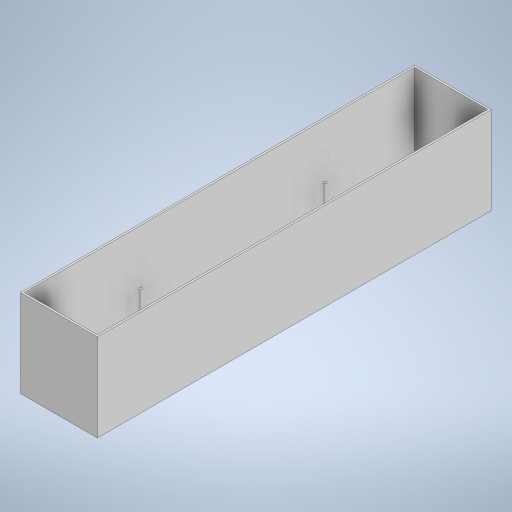
# Autodesk Inventor part: Box
Saved by Autodesk Inventor 2023 (Build 270158030, 158C)
## iProperties
Created: 2023-02-14
Part Number: Box
Material: Generic
Document SubType Name: Modeling
Designer: jeremyy
Density: 1 g/cm^3
Appearance: Default
Author: jeremyy
Autodesk Inventor part; units mm, degrees
ref_plane "YZ Plane" through (0, 0, 0) normal (1, 0, 0) x (0, 1, 0)
ref_plane "XZ Plane" through (0, 0, 0) normal (0, 1, 0) x (-1, 0, 0)
ref_plane "XY Plane" through (0, 0, 0) normal (0, 0, 1) x (1, 0, 0)
sketch "Sketch1" plane through (0, 0, 0) normal (0, 1, 0) x (-1, 0, 0)
  line L0 (0, 0) -> (127, 0)
  line L1 (127, 0) -> (127, -651.51)
  line L2 (127, -651.51) -> (0, -651.51)
  line L3 (0, -651.51) -> (0, 0)
  line L4 (123.825, -3.175) -> (3.175, -3.175)
  line L5 (3.175, -3.175) -> (3.175, -648.335)
  line L6 (3.175, -648.335) -> (123.825, -648.335)
  line L7 (123.825, -648.335) -> (123.825, -3.175)
  circle A0 centre (101.6, -478.155) radius 2.3812
  circle A1 centre (25.4, -478.155) radius 2.3813
  line L8 (3.175, -325.755) -> (14.531, -325.755)
  circle A2 centre (101.6, -173.355) radius 2.3812
  circle A3 centre (25.4, -173.355) radius 2.3813
  dimension "d0" = 127
  dimension "d1" = 651.51
  dimension "d2" = 3.175
  dimension "d13" = 4.7625
  dimension "d14" = 4.7625
  dimension "d15" = 76.2
  dimension "d16" = 25.4
  dimension "d17" = 152.4
  constraints: 18 end point, 4 centre point, 4 parallel, 2 horizontal, 2 perpendicular, 2 symmetric about line, 1 midpoint, 5 other
  measures "d0" distance of L1.end L2.end
  measures "d1" distance of L0.end L1.end
  measures "d2" distance between parallel lines of L0 L4
  measures "d13" diameter of A0
  measures "d14" diameter of A1
  measures "d15" distance of A1.centre A0.centre
  measures "d16" distance from line of A1.centre L3
  measures "d17" distance from line of L8 A1.centre
extrude "Extrusion1" add sketch "Sketch1" along normal blind 3.175 contours L7 L6 L5 L4
extrude "Extrusion2" add sketch "Sketch1" along normal blind 144.78 contours L0 L1 L2 L3
sketch "Sketch2" plane through (0, 0, 0) normal (0, -1, 0) x (1, 0, 0)
  line L0 (-50.8, -76.2) -> (-76.2, -76.2)
  line L1 (-76.2, -76.2) -> (-76.2, -88.9)
  line L2 (-76.2, -88.9) -> (-50.8, -88.9)
  line L3 (-50.8, -88.9) -> (-50.8, -76.2)
  line L4 (0, 0) -> (0, -651.51) projected
  line L5 (0, -325.755) -> (-127, -325.755)
  line L6 (-127, -651.51) -> (-127, 0) projected
  line L7 (-50.8, -575.31) -> (-76.2, -575.31)
  line L8 (-76.2, -575.31) -> (-76.2, -562.61)
  line L9 (-76.2, -562.61) -> (-50.8, -562.61)
  line L10 (-50.8, -562.61) -> (-50.8, -575.31)
  line L11 (-127, 0) -> (0, 0) projected
  dimension "d7" = 25.4
  dimension "d8" = 12.7
  dimension "d9" = 50.8
  dimension "d10" = 76.2
  constraints: 18 end point, 4 symmetric about line, 2 midpoint, 2 parallel, 1 horizontal, 1 perpendicular
  measures "d7" distance of L2.end L1.end
  measures "d8" distance of L1.end L0.end
  measures "d9" distance between parallel lines of L4 L3
  measures "d10" distance between parallel lines of L11 L0
extrude "Extrusion3" add sketch "Sketch2" along normal blind 12.7 contours L3 L2 L1 L0 | L7 L8 L9 L10
extrude "Extrusion4" add sketch "Sketch1" along normal blind 76.2 contours A0 | A1 | A2 | A3
sketch "Sketch3" plane through (0, 3.175, 0) normal (0, 1, 0) x (1, 0, 0)
  line L0 (-3.175, 3.175) -> (-3.175, 648.335) projected
  line L1 (-123.825, 648.335) -> (-123.825, 3.175) projected
  line L2 (-3.175, 66.675) -> (-123.825, 66.675)
  line L3 (-123.825, 66.675) -> (-123.825, 117.475)
  line L4 (-123.825, 117.475) -> (-3.175, 117.475)
  line L5 (-3.175, 117.475) -> (-3.175, 66.675)
  line L6 (-3.175, 3.175) -> (-123.825, 3.175) projected
  line L7 (-127, 651.51) -> (-127, 0) projected
  line L8 (-127, 325.755) -> (-116.0264, 325.755)
  line L9 (-3.175, 584.835) -> (-123.825, 584.835)
  line L10 (-123.825, 584.835) -> (-123.825, 534.035)
  line L11 (-123.825, 534.035) -> (-3.175, 534.035)
  line L12 (-3.175, 534.035) -> (-3.175, 584.835)
  point P0 (0, 0)
  point P1 (-3.175, 534.035)
  point P2 (-3.175, 117.475)
  dimension "d20" = 50.8
  dimension "d21" = 63.5
  constraints: 18 end point, 4 symmetric about line, 2 horizontal, 2 parallel, 2 point on line, 1 midpoint, 1 perpendicular
  measures "d20" distance between parallel lines of L4 L2
  measures "d21" distance between parallel lines of L6 L2
extrude "Extrusion5" add sketch "Sketch3" along normal blind 19.05 contours L2 L1 L4 L0 | L11 L1 L9 L0
body "Solid1"
